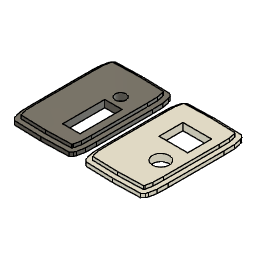
NeoDK-Covers v4 (Autodesk Fusion 360 design; units mm, degrees)
Autodesk Fusion 360 part; units mm, degrees
sketch "cover" plane through (0, 0, 0) normal (0, 1, 0) x (1, 0, 0)
  line L0 (13.5, -21.5) -> (-13.5, -21.5) construction
  line L1 (-13.5, -21.5) -> (-13.5, 21.5) construction
  line L2 (-13.5, 21.5) -> (13.5, 21.5) construction
  line L3 (13.5, 21.5) -> (13.5, -21.5) construction
  line L4 (13.5, -21.5) -> (-13.5, 21.5) construction
  line L5 (-13.5, -21.5) -> (13.5, 21.5) construction
  line L6 (0, 21.5) -> (11.4729, 21.1591)
  line L7 (11.4729, 21.1591) -> (12.4104, 20.2086)
  line L8 (12.4104, 20.2086) -> (12.7846, 19.2784)
  line L9 (12.7846, 19.2784) -> (13.392, 16.1994)
  line L10 (13.392, 16.1994) -> (13.5, 11.6878)
  line L11 (13.5, 11.6878) -> (13.5, 0)
  line L12 (2.5, 0) -> (20, 0)
  line L13 (13.392, -16.1994) -> (13.5, -11.6878)
  line L14 (12.7846, -19.2784) -> (13.392, -16.1994)
  line L15 (11.4729, -21.1591) -> (12.4104, -20.2086)
  line L16 (12.4104, -20.2086) -> (12.7846, -19.2784)
  line L17 (0, -21.5) -> (11.4729, -21.1591)
  line L18 (13.5, -11.6878) -> (13.5, 0)
  line L19 (0, -20) -> (0, -2.5)
  line L20 (0, 21.5) -> (-11.4729, 21.1591)
  line L21 (-11.4729, 21.1591) -> (-12.4104, 20.2086)
  line L22 (-12.7846, 19.2784) -> (-13.392, 16.1994)
  line L23 (-12.4104, 20.2086) -> (-12.7846, 19.2784)
  line L24 (-13.392, 16.1994) -> (-13.5, 11.6878)
  line L25 (-13.5, 11.6878) -> (-13.5, 0)
  line L26 (-13.5, -11.6878) -> (-13.5, 0)
  line L27 (-13.392, -16.1994) -> (-13.5, -11.6878)
  line L28 (-12.7846, -19.2784) -> (-13.392, -16.1994)
  line L29 (-12.4104, -20.2086) -> (-12.7846, -19.2784)
  line L30 (-11.4729, -21.1591) -> (-12.4104, -20.2086)
  line L31 (0, -21.5) -> (-11.4729, -21.1591)
  line L32 (11.5, -11.6638) -> (11.5, 0)
  line L33 (11.5, 11.6638) -> (11.5, 0)
  line L34 (11.3967, 15.9803) -> (11.5, 11.6638)
  line L35 (10.8588, 18.7066) -> (11.3967, 15.9803)
  line L36 (10.7046, 19.0899) -> (10.8588, 18.7066)
  line L37 (10.612, 19.1838) -> (10.7046, 19.0899)
  line L38 (0, 19.4991) -> (10.612, 19.1838)
  line L39 (0, 19.4991) -> (-10.612, 19.1838)
  line L40 (-10.612, 19.1838) -> (-10.7046, 19.0899)
  line L41 (-10.7046, 19.0899) -> (-10.8588, 18.7066)
  line L42 (-10.8588, 18.7066) -> (-11.3967, 15.9803)
  line L43 (-11.3967, 15.9803) -> (-11.5, 11.6638)
  line L44 (-11.5, 11.6638) -> (-11.5, 0)
  line L45 (-11.5, -11.6638) -> (-11.5, 0)
  line L46 (-11.3967, -15.9803) -> (-11.5, -11.6638)
  line L47 (-10.8588, -18.7066) -> (-11.3967, -15.9803)
  line L48 (-10.7046, -19.0899) -> (-10.8588, -18.7066)
  line L49 (-10.612, -19.1838) -> (-10.7046, -19.0899)
  line L50 (0, -19.4991) -> (-10.612, -19.1838)
  line L51 (0, -19.4991) -> (10.612, -19.1838)
  line L52 (10.612, -19.1838) -> (10.7046, -19.0899)
  line L53 (10.7046, -19.0899) -> (10.8588, -18.7066)
  line L54 (10.8588, -18.7066) -> (11.3967, -15.9803)
  line L55 (11.3967, -15.9803) -> (11.5, -11.6638)
  dimension "d1" = 27
  dimension "d2" = 43
  dimension "d3" = -2
  constraint horizontal L0
  constraint perpendicular L0 L1
  constraint parallel L0 L2
  constraint parallel L1 L3
  constraint coincident L4 origin
  constraint coincident L5 origin
  constraint midpoint L2 L6.start
  constraint coincident L3 L10.end
  constraint midpoint L3 L11.end
  constraint symmetric L6.start L12 L17.start
  constraint symmetric L6.end L12 L15.start
  constraint symmetric L7.end L12 L15.end
  constraint symmetric L8.end L12 L14.start
  constraint symmetric L9.end L12 L13.start
  constraint symmetric L10.end L12 L13.end
  constraint symmetric L11.end L12 L18.end
  constraint symmetric L6.start L19 L20.start
  constraint symmetric L6.end L19 L20.end
  constraint symmetric L7.end L19 L21.end
  constraint symmetric L8.end L19 L22.start
  constraint symmetric L9.end L19 L22.end
  constraint symmetric L10.end L19 L24.end
  constraint symmetric L11.end L19 L25.end
  constraint symmetric L13.start L19 L27.start
  constraint symmetric L13.end L19 L26.start
  constraint symmetric L14.start L19 L28.start
  constraint symmetric L15.start L19 L30.start
  constraint symmetric L15.end L19 L29.start
  constraint symmetric L17.start L19 L31.start
  measures "d1" distance of L1.end L2.end
  measures "d2" distance of L0.end L1.end
extrude "Extrude2" add sketch "cover" along normal blind 3 contours L32 L33 L34 L35 L36 L37 L38 L39 L40 L41 L42 L43 L44 L45 L46 L47 L48 L49 L50 L51 L52 L53 L54 L55 makes body 1
extrude "Extrude1" add sketch "cover" along normal blind 1.6 contours L6 L7 L8 L9 L10 L11 L13 L14 L15 L16 L17 L18 L20 L21 L22 L23 L24 L25 L26 L27 L28 L29 L30 L31 | L32 L33 L34 L35 L36 L37 L38 L39 L40 L41 L42 L43 L44 L45 L46 L47 L48 L49 L50 L51 L52 L53 L54 L55 bodies 1
sketch "rear-holes" plane through (0, 0, 0) normal (0, 1, 0) x (1, 0, 0)
  line L0 (-4, 2) -> (8, 2)
  line L1 (8, 2) -> (8, 12)
  line L2 (8, 12) -> (-4, 12)
  line L3 (-4, 12) -> (-4, 2)
  circle A0 centre (5.0661, -6.3322) radius 3.5
  dimension "d8" = 7
  constraint horizontal L0
  constraint vertical L1
  constraint horizontal L2
  constraint vertical L3
  measures "d8" diameter of A0
copy_body "CopyPasteBodies1" bodies 1 makes body 2
move_body "Move1" bodies 2 to x (1, 0, 0) y (0, 1, 0) z (0, 0, 1) at (0, 0, 0)
extrude "Extrude3" cut sketch "rear-holes" along normal through all bodies 1
sketch "front-holes" plane through (0, 0, 0) normal (0, 1, 0) x (1, 0, 0)
  circle A0 centre (3.7055, 8.2093) radius 2.25
  line L0 (1.284, 3.982) -> (8.5455, 3.982)
  line L1 (8.5455, 3.982) -> (8.5455, -13.649)
  line L2 (8.5455, -13.649) -> (1.284, -13.649)
  line L3 (1.284, -13.649) -> (1.284, 3.982)
  dimension "d12" = 4.5
  constraint horizontal L0
  constraint vertical L1
  constraint horizontal L2
  constraint vertical L3
  measures "d12" diameter of A0
copy_body "CopyPasteBodies2" bodies 2 makes body 3
move_body "Move2" bodies 3 to x (1, 0, 0) y (0, 1, 0) z (0, 0, 1) at (0, 0, 0)
extrude "Extrude4" cut sketch "front-holes" along normal through all bodies 3
move_body "Move3" bodies 1 to x (1, 0, 0) y (0, 1, 0) z (0, 0, 1) at (30, 0, 0)
hidden bodies 2
named bodies: "Cover-Rear", "Whole-Cover", "Cover-Stock", "Cover-Front"
